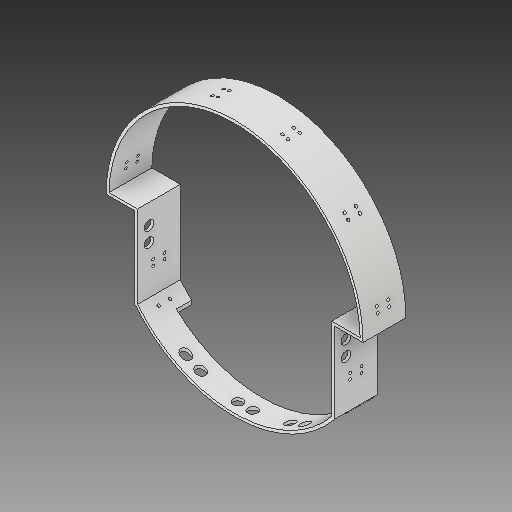
# Autodesk Inventor part: CW000
Saved by Autodesk Inventor 2017 SP1 (Build 210196100, 196)
## iProperties
Created: 2017-05-15
Part Number: CW000
Material: ABS Plastic
Document SubType Name: Modeling
Designer: zallen
Density: 1.06 g/cm^3
Appearance: Smooth - White
Author: zallen
Autodesk Inventor part; units mm, degrees
ref_plane "YZ Plane" through (0, 0, 0) normal (1, 0, 0) x (0, 1, 0)
ref_plane "XZ Plane" through (0, 0, 0) normal (0, 1, 0) x (-1, 0, 0)
ref_plane "XY Plane" through (0, 0, 0) normal (0, 0, 1) x (1, 0, 0)
sketch "Sketch1" plane through (0, 0, 0) normal (0, 0, 1) x (1, 0, 0)
  line L0 (-225, 0) -> (-175, 0) construction
  line L1 (-175, 0) -> (-175, -141.4214) construction
  line L2 (225, 0) -> (175, 0) construction
  line L3 (175, 0) -> (175, -141.4214) construction
  arc A0 (225, 0) -> (-225, 0) centre (0, 0) ccw
  arc A1 (-175, -141.4214) -> (175, -141.4214) centre (0, 0) ccw
  line L4 (-225, 0) -> (-175, 0)
  line L5 (-175, -141.4214) -> (-175, 0)
  line L6 (225, 0) -> (175, 0)
  line L7 (175, -141.4214) -> (175, 0)
  arc A2 (219.9432, 5) -> (-219.9432, 5) centre (0, 0) ccw
  line L8 (219.9432, 5) -> (170, 5)
  line L9 (170, 5) -> (170, -139.6424)
  arc A3 (-170, -139.6424) -> (170, -139.6424) centre (0, 0) ccw
  line L10 (-170, -139.6424) -> (-170, 5)
  line L11 (-170, 5) -> (-219.9432, 5)
  dimension "d1" = 50
  dimension "d2" = 50
  dimension "d3" = 5
  constraints: 24 end point, 8 point on circle, 4 centre point, 4 perpendicular, 3 collinear, 2 horizontal, 5 other
  measures "d1" distance of L0.start L0.end
  measures "d2" distance of L2.start L2.end
  measures "d3" radial gap between concentric circles of A0 A2
extrude "Extrusion1" add sketch "Sketch1" along normal blind 75
sketch "Sketch3" plane through (-175, -141.4214, 0) normal (-1, 0, 0) x (0, 0, 1)
  circle A0 centre (47.5, 46.6338) radius 2.5 projected
  circle A1 centre (47.5, 56.6338) radius 2.5 projected
  circle A2 centre (27.5, 56.6338) radius 2.5 projected
  circle A3 centre (27.5, 46.6338) radius 2.5 projected
  circle A4 centre (47.5, 46.6338) radius 2.5
  circle A5 centre (47.5, 56.6338) radius 2.5
  circle A6 centre (27.5, 56.6338) radius 2.5
  circle A7 centre (27.5, 46.6338) radius 2.5
  point P0 (0, 141.4214)
  constraints: 4 centre point, 4 coincident, 4 concentric
extrude "Extrusion2" cut sketch "Sketch3" against normal through all
ref_plane "Work Plane1" through (297.5736, -480.0674, 65.4771) normal (0.9880034, 0.154432, 0) x (0.0420373, -0.2689403, 0.9622391)
sketch "Sketch4" plane through (297.5736, -480.0674, 65.4771) normal (0.9880034, 0.154432, 0) x (0.0420373, -0.2689403, 0.9622391)
  circle A0 centre (-157.5559, -490.9128) radius 2.5 projected
  circle A1 centre (-160.278, -500.5352) radius 2.5 projected
  circle A2 centre (-176.8007, -485.4687) radius 2.5 projected
  circle A3 centre (-179.5227, -495.0911) radius 2.5 projected
  circle A4 centre (-157.5559, -490.9128) radius 2.5
  circle A5 centre (-160.278, -500.5352) radius 2.5
  circle A6 centre (-176.8007, -485.4687) radius 2.5
  circle A7 centre (-179.5227, -495.0911) radius 2.5
  point P0 (-204.6233, -482.7942)
  constraints: 4 centre point, 4 coincident, 4 concentric
extrude "Extrusion3" cut sketch "Sketch4" along normal through all
ref_plane "Work Plane2" through (324.8264, -34.8132, -10) normal (0.7480036, 0.6636947, 0) x (0, 0, -1)
sketch "Sketch5" plane through (324.8264, -34.8132, -10) normal (0.7480036, 0.6636947, 0) x (0, 0, -1)
  circle A0 centre (-57.5, 236.626) radius 2.5 projected
  circle A1 centre (-57.5, 246.626) radius 2.5 projected
  circle A2 centre (-37.5, 236.626) radius 2.5 projected
  circle A3 centre (-37.5, 246.626) radius 2.5 projected
  circle A4 centre (-57.5, 236.626) radius 2.5
  circle A5 centre (-57.5, 246.626) radius 2.5
  circle A6 centre (-37.5, 236.626) radius 2.5
  circle A7 centre (-37.5, 246.626) radius 2.5
  point P0 (-10, 241.626)
  constraints: 4 centre point, 4 coincident, 4 concentric
extrude "Extrusion4" cut sketch "Sketch5" along normal through all
ref_plane "Work Plane3" through (-106.4712, 258.6929, 719.0942) normal (0.2726306, 0.9621188, 0) x (-0.8394563, 0.2378723, 0.4885999)
sketch "Sketch6" plane through (-106.4712, 258.6929, 719.0942) normal (0.2726306, 0.9621188, 0) x (-0.8394563, 0.2378723, 0.4885999)
  circle A0 centre (-483.4173, -499.0173) radius 2.5 projected
  circle A1 centre (-474.6922, -503.9033) radius 2.5 projected
  circle A2 centre (-493.1893, -516.4675) radius 2.5 projected
  line L0 (-502.2632, -542.9044) -> (-465.6182, -477.4663) projected
  circle A3 centre (-484.4642, -521.3535) radius 2.5 projected
  line L1 (-502.2632, 0) -> (-465.6182, 0) projected
  circle A4 centre (-483.4173, -499.0173) radius 2.5
  circle A5 centre (-474.6922, -503.9033) radius 2.5
  circle A6 centre (-484.4642, -521.3535) radius 2.5
  circle A7 centre (-493.1893, -516.4675) radius 2.5
  constraints: 4 centre point, 4 coincident, 4 concentric
extrude "Extrusion5" cut sketch "Sketch6" along normal through all
ref_plane "Work Plane4" through (-1107.3415, -85.2588, 510.2398) normal (-0.2726306, 0.9621188, 0) x (0.3789755, 0.1073883, -0.9191547)
sketch "Sketch7" plane through (-1107.3415, -85.2588, 510.2398) normal (-0.2726306, 0.9621188, 0) x (0.3789755, 0.1073883, -0.9191547)
  circle A0 centre (852.1711, -813.7595) radius 2.5 projected
  circle A1 centre (856.11, -822.951) radius 2.5 projected
  circle A2 centre (874.4931, -815.0731) radius 2.5 projected
  circle A3 centre (870.5542, -805.8815) radius 2.5 projected
  circle A4 centre (852.1711, -813.7595) radius 2.5
  circle A5 centre (870.5542, -805.8815) radius 2.5
  circle A6 centre (874.4931, -815.0731) radius 2.5
  circle A7 centre (856.11, -822.951) radius 2.5
  point P0 (897.8004, -799.6451)
  constraints: 4 centre point, 4 coincident, 4 concentric
extrude "Extrusion6" cut sketch "Sketch7" along normal through all
ref_plane "Work Plane5" through (-206.3107, 98.7576, 14.764) normal (-0.7480036, 0.6636947, 0) x (-0.3715569, -0.4187557, 0.8286067)
sketch "Sketch8" plane through (-206.3107, 98.7576, 14.764) normal (-0.7480036, 0.6636947, 0) x (-0.3715569, -0.4187557, 0.8286067)
  circle A0 centre (-10.9747, 74.7185) radius 2.5 projected
  circle A1 centre (-5.3764, 66.4325) radius 2.5 projected
  circle A2 centre (-21.9485, 55.2358) radius 2.5 projected
  circle A3 centre (-27.5469, 63.5219) radius 2.5 projected
  circle A4 centre (-5.3764, 66.4325) radius 2.5
  circle A5 centre (-21.9485, 55.2358) radius 2.5
  circle A6 centre (-27.5469, 63.5219) radius 2.5
  circle A7 centre (-10.9747, 74.7185) radius 2.5
  point P0 (-47.5344, 43.9835)
  constraints: 4 centre point, 4 coincident, 4 concentric
extrude "Extrusion7" cut sketch "Sketch8" along normal through all
ref_plane "Work Plane6" through (-203.409, 122.366, 1080.5241) normal (-0.9880034, 0.154432, 0) x (-0.1515994, -0.9698817, 0.190649)
sketch "Sketch9" plane through (-203.409, 122.366, 1080.5241) normal (-0.9880034, 0.154432, 0) x (-0.1515994, -0.9698817, 0.190649)
  circle A0 centre (-114.0095, -1030.1837) radius 2.5 projected
  circle A1 centre (-104.1929, -1032.0902) radius 2.5 projected
  circle A2 centre (-117.8224, -1049.8169) radius 2.5 projected
  circle A3 centre (-108.0059, -1051.7234) radius 2.5 projected
  circle A4 centre (-104.1929, -1032.0902) radius 2.5
  circle A5 centre (-108.0059, -1051.7234) radius 2.5
  circle A6 centre (-117.8224, -1049.8169) radius 2.5
  circle A7 centre (-114.0095, -1030.1837) radius 2.5
  point P0 (-118.157, -1077.7657)
  constraints: 4 centre point, 4 coincident, 4 concentric
extrude "Extrusion8" cut sketch "Sketch9" along normal through all
ref_plane "Work Plane7" through (-558.1067, 254.5703, 43.9955) normal (-0.7135281, -0.7006267, 0) x (-0.1739901, 0.177194, 0.9686742)
sketch "Sketch10" plane through (-558.1067, 254.5703, 43.9955) normal (-0.7135281, -0.7006267, 0) x (-0.1739901, 0.177194, 0.9686742)
  circle A0 centre (-137.5769, -550.7552) radius 2.5 projected
  circle A1 centre (-156.9504, -545.7885) radius 2.5 projected
  circle A2 centre (-137.5769, -550.7552) radius 2.5
  circle A3 centre (-156.9504, -545.7885) radius 2.5
  point P0 (-184.8306, -543.8026)
  constraints: 2 centre point, 2 coincident, 2 concentric
extrude "Extrusion9" cut sketch "Sketch10" along normal through all
ref_plane "Work Plane8" through (107.3441, -311.532, 65) normal (0.9459555, -0.3242964, 0) x (0, 0, -1)
sketch "Sketch11" plane through (107.3441, -311.532, 65) normal (0.9459555, -0.3242964, 0) x (0, 0, -1)
  circle A0 centre (17.5, 173.6211) radius 2.5 projected
  circle A1 centre (37.5, 173.6211) radius 2.5 projected
  circle A2 centre (17.5, 173.6211) radius 2.5
  circle A3 centre (37.5, 173.6211) radius 2.5
  point P0 (65, 259.8841)
  constraints: 2 centre point, 2 coincident, 2 concentric
extrude "Extrusion10" cut sketch "Sketch11" along normal through all
ref_plane "Work Plane9" through (-170, -139.6424, 0) normal (0.0051563, 0.9999867, 0) x (0, 0, 1)
sketch "Sketch12" plane through (-170, -139.6424, 0) normal (0.0051563, 0.9999867, 0) x (0, 0, 1)
  line L0 (0, 0) -> (0, 339.9955) projected
  line L1 (0, 20) -> (27, 20)
  line L2 (27, 20) -> (27, 320)
  line L3 (27, 320) -> (0, 320)
  line L4 (0, 320) -> (0, 20)
  point P0 (0, 169.2777)
  dimension "d24" = 27
  dimension "d25" = 20
  dimension "d26" = 300
  constraints: 8 end point, 2 parallel, 1 horizontal, 1 perpendicular, 1 point on line
  measures "d24" distance of L3.end L2.end
  measures "d25" distance from line of L0.start L1
  measures "d26" distance of L1.end L2.end
extrude "Extrusion11" cut sketch "Sketch12" against normal through all
sketch "Sketch13" plane through (175, -141.4214, 0) normal (1, 0, 0) x (0, 0, -1)
  circle A0 centre (-55, 85.4214) radius 8.5
  circle A1 centre (-55, 111.4214) radius 8.5
  line L0 (0, 141.4214) -> (0, 0) projected
  line L1 (0, 141.4214) -> (-75, 141.4214) projected
  dimension "d29" = 17
  dimension "d30" = 17
  dimension "d31" = 26
  dimension "d32" = 55
  dimension "d35" = 30
  constraints: 2 centre point, 1 vertical alignment
  measures "d29" diameter of A0
  measures "d30" diameter of A1
  measures "d31" distance of A1.centre A0.centre
  measures "d32" distance from line of L0 A0.centre
  measures "d35" distance from line of L1 A1.centre
extrude "Extrusion12" cut sketch "Sketch13" against normal through all
sketch "Sketch14" plane through (-170, -139.6424, 0) normal (0.0051563, 0.9999867, 0) x (0, 0, 1)
  circle A0 centre (55, 64.7777) radius 8.5
  circle A1 centre (55, 90.7777) radius 8.5
  circle A2 centre (55, 247.7777) radius 8.5
  circle A3 centre (55, 273.7777) radius 8.5
  circle A4 centre (55, 156.2777) radius 8.5
  circle A5 centre (55, 182.2777) radius 8.5
  point P0 (0, 169.2777)
  dimension "d36" = 17
  dimension "d37" = 17
  dimension "d38" = 26
  dimension "d39" = 17
  dimension "d40" = 17
  dimension "d41" = 26
  dimension "d45" = 17
  dimension "d46" = 17
  dimension "d47" = 26
  dimension "d49" = 13
  dimension "d50" = 65.5
  dimension "d51" = 65.5
  dimension "d52" = 55
  constraints: 6 centre point, 5 vertical alignment
  measures "d36" diameter of A0
  measures "d37" diameter of A1
  measures "d38" distance of A1.centre A0.centre
  measures "d39" diameter of A2
  measures "d40" diameter of A3
  measures "d41" distance of A3.centre A2.centre
  measures "d45" diameter of A4
  measures "d46" diameter of A5
  measures "d47" distance of A5.centre A4.centre
  measures "d49" vertical distance of point (0, 169.278) A4.centre
  measures "d50" distance of A4.centre A1.centre
  measures "d51" distance of A2.centre A5.centre
  measures "d52" horizontal distance of point (0, 169.278) A2.centre
extrude "Extrusion13" cut sketch "Sketch14" against normal through all
body "Solid1"
